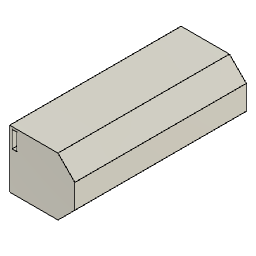
SandPolisher_3rdTry v12 (Autodesk Fusion 360 archive; units mm, degrees)
design "RobotisBatt"
Autodesk Fusion 360 part; units mm, degrees
sketch "Sketch1" plane through (0, 0, 0) normal (1, 0, 0) x (0, 1, 0) in component "RobotisBatt"
  line L0 (0, 0) -> (71, 0)
  line L1 (71, 0) -> (71, 24)
  line L2 (71, 24) -> (0, 24)
  line L3 (0, 24) -> (0, 0)
  dimension "d1" = 71
  dimension "d2" = 24
  constraint horizontal L0
  constraint vertical L1
  constraint horizontal L2
  constraint vertical L3
  constraint coincident L0.start L3.end
  measures "d1" distance of L1.end L2.end
  measures "d2" distance of L0.start L2.end
extrude "Extrude1" add sketch "Sketch1" along normal blind 27 in component "RobotisBatt"
chamfer "Chamfer1" distance 7 angle 45 2 edges at (27, 35.5, 24) (27, 35.5, 0) in component "RobotisBatt"
sketch "Sketch2" plane through (0, 0, 0) normal (0, -1, 0) x (1, 0, 0) in component "RobotisBatt"
  line L0 (20, 0) -> (27, 7)
  line L1 (27, 7) -> (27, 17)
  line L2 (27, 17) -> (20, 24)
  line L3 (20, 24) -> (0, 24)
  line L4 (0, 24) -> (0, 0)
  line L5 (0, 0) -> (20, 0)
  line L6 (1, 23) -> (3, 23)
  line L7 (3, 23) -> (3, 16)
  line L8 (3, 16) -> (1, 16)
  line L9 (1, 16) -> (1, 23)
  constraint horizontal L6
  constraint vertical L7
  constraint horizontal L8
  constraint vertical L9
extrude "Extrude2" cut sketch "Sketch2" against normal blind 4 contours L6 L7 L8 L9 in component "RobotisBatt"
component "RobotisBatt" placed x (1, 0, 0) y (0, 1, 0) z (0, 0, 1) at (0, 0, 0)
